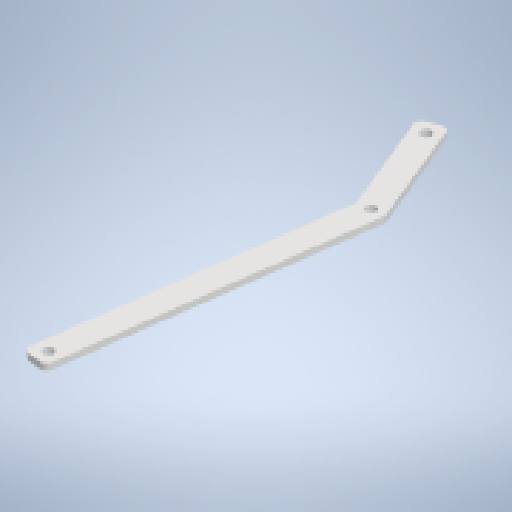
# Autodesk Inventor part: PB IN
Saved by Autodesk Inventor 2023 (Build 270158000, 158)
## iProperties
Created: 2023-03-01
Part Number: PB IN
Material: Generic
Document SubType Name: Modeling
Designer: Gabriel - T3 CAD
Density: 1 g/cm^3
Appearance: Default
Author: Gabriel - T3 CAD
Autodesk Inventor part; units mm, degrees
ref_plane "YZ Plane" through (0, 0, 0) normal (1, 0, 0) x (0, 1, 0)
ref_plane "XZ Plane" through (0, 0, 0) normal (0, 1, 0) x (-1, 0, 0)
ref_plane "XY Plane" through (0, 0, 0) normal (0, 0, 1) x (1, 0, 0)
sketch "Sketch1" plane through (0, 0, 0) normal (0, 1, 0) x (-1, 0, 0)
  line L0 (0, 0) -> (0, 190.5)
  line L1 (0, 190.5) -> (-19.3142, 47.0141)
  line L2 (-19.3142, 47.0141) -> (0, 0)
  line L3 (8.2867, -3.4607) -> (-3.4607, -8.2867)
  line L4 (-3.4607, -8.2867) -> (-25.8344, 46.1749)
  line L5 (-25.8344, 46.1749) -> (-14.0871, 51.0009)
  line L6 (-14.0871, 51.0009) -> (8.2867, -3.4607)
  line L7 (-5.4461, 197.6404) -> (7.1404, 195.9461)
  line L8 (7.1404, 195.9461) -> (-13.2479, 44.4807)
  line L9 (-13.2479, 44.4807) -> (-25.8344, 46.1749)
  line L10 (-25.8344, 46.1749) -> (-5.4461, 197.6404)
  circle A0 centre (0, 0) radius 2.5797
  circle A1 centre (-19.3142, 47.0141) radius 2.5797
  circle A2 centre (0, 190.5) radius 2.5797
  point P0 (0.8471, 196.7932)
  point P1 (2.413, -5.8737)
  point P2 (-12.7939, 47.8532)
  dimension "d0" = 150
  dimension "d1" = 190.5
  dimension "d2" = 144.78
  dimension "d3" = 12.7
  dimension "d4" = 5.1594
  dimension "d5" = 6.35
  dimension "d6" = 6.35
  constraints: 22 end point, 6 parallel, 4 coincident, 4 point on line, 3 centre point, 2 equal radius, 2 midpoint, 2 perpendicular, 1 equal length, 1 vertical
  measures "d0" angle of L2 L1
  measures "d1" distance of L0.start L0.end
  measures "d2" distance of L0.end L1.end
  measures "d3" distance of L3.start L3.end
  measures "d4" diameter of A0
  measures "d5" distance from line of L0.end L7
  measures "d6" distance from line of point (0, 0) L3
extrude "Extrusion1" add sketch "Sketch1" along normal blind 3.175 contours A0 L2 A1 L9 L8 L6 L0 | L0 L6 L3 L4 L9 A1 L2 A0 | A1 L9 L2 | L2 L9 A1 | L8 L6 L5 A1 L1 A2 L0 | L0 A2 L1 A1 L5 L10 L7 L8 | L8 L9 A1 L5 L6 | L9 A1 L5 L1 L2 | L2 L1 L5 A1 L9 | L9 L5 A1 | A1 L1 L5 | L5 L1 A1
fillet "Fillet1" radius 3.175 6 edges at (-7.1404, 1.5875, 195.9461) (5.4461, 1.5875, 197.6404) (25.8344, 1.5875, 46.1749) (12.7939, 1.5875, 47.8532) (3.4607, 1.5875, -8.2867) (-8.2867, 1.5875, -3.4607)
body "Solid1"
